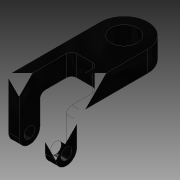
# Autodesk Inventor part: Piston_Holder
Saved by Autodesk Inventor 2015 (Build 190159000, 159)
## iProperties
Created: 2017-02-21
Part Number: Piston_Holder
Material: Acetal Resin, Black
Document SubType Name: Modeling
Designer: Guy
Density: 1.425 g/cm^3
Appearance: Smooth - Black
Author: Guy
Autodesk Inventor part; units mm, degrees
ref_plane "YZ Plane" through (0, 0, 0) normal (1, 0, 0) x (0, 1, 0)
ref_plane "XZ Plane" through (0, 0, 0) normal (0, 1, 0) x (-1, 0, 0)
ref_plane "XY Plane" through (0, 0, 0) normal (0, 0, 1) x (1, 0, 0)
sketch "Sketch1" plane through (0, 0, 0) normal (0, 0, 1) x (1, 0, 0)
  circle A0 centre (0, 0) radius 5
  circle A1 centre (0, 0) radius 9
  line L0 (-9, 0) -> (-9, -35)
  line L1 (9, 0) -> (9, -35)
  line L2 (0, 0) -> (0, -54.7816)
  line L3 (-9, -35) -> (-5, -35)
  line L4 (-5, -35) -> (-5, -15)
  line L5 (5, -15) -> (5, -35)
  line L6 (5, -35) -> (9, -35)
  line L7 (-5, -15) -> (5, -15)
  dimension "d0" = 10
  dimension "d1" = 18
  dimension "d4" = 15
  dimension "d6" = 20
  dimension "d22" = 4
  dimension "d23" = 4
  constraints: 16 end point, 3 coincident, 2 centre point, 2 horizontal, 2 parallel, 2 point on circle, 2 tangent, 1 collinear, 1 perpendicular, 1 point on line, 1 vertical
  measures "d0" diameter of A0
  measures "d1" diameter of A1
  measures "d4" distance from line of L7 point (0, 0)
  measures "d6" distance between parallel lines of L3 L7
  measures "d22" distance between parallel lines of L1 L5
  measures "d23" distance between parallel lines of L0 L4
extrude "Extrusion1" add sketch "Sketch1" along normal blind 23 contours A0 | A1 | L1 L6 L5 L7 L2 A1 | A1 L2 L7 L4 L3 L0
sketch "Sketch2" plane through (9, -35, 0) normal (1, 0, 0) x (0, 0, -1)
  circle A0 centre (-4, 4) radius 2.1
  line L0 (0, 0) -> (0, 35) projected
  line L1 (0, 35) -> (-23, 35) projected
  line L2 (-23, 0) -> (-23, 35) projected
  line L3 (0, 0) -> (-23, 0) projected
  dimension "d9" = 4.2
  dimension "d10" = 4
  dimension "d20" = 4
  constraints: 1 centre point
  measures "d9" diameter of A0
  measures "d10" distance from line of L3 A0.centre
  measures "d20" distance from line of L0 A0.centre
extrude "Extrusion2" cut sketch "Sketch2" against normal through all contours A0
fillet "Fillet1" radius 2 2 edges at (-5, -15, 11.5) (5, -15, 11.5)
sketch "Sketch5" plane through (9, -35, 0) normal (1, 0, 0) x (0, 0, -1)
  circle A0 centre (-4, 4) radius 2.1 projected
  line L0 (0, 0) -> (0, 35) projected
  line L1 (0, 35) -> (-23, 35) projected
  line L2 (-23, 0) -> (-23, 35) projected
  line L3 (0, 0) -> (-23, 0) projected
  line L4 (-23, 20) -> (0, 20) projected
  line L5 (0, 20) -> (-23, 20) projected
  line L6 (-15, 8) -> (0, 8)
  line L7 (0, 8) -> (0, 53.1691)
  line L8 (0, 53.1691) -> (-15, 53.1691)
  line L9 (-15, 53.1691) -> (-15, 8)
  line L10 (0, 0) -> (0, 35) projected
  line L11 (0, 35) -> (0, 35) projected
  line L12 (0, 35) -> (-23, 35) projected
  line L13 (-23, 35) -> (-23, 35) projected
  line L14 (0, 35) -> (-23, 35) projected
  dimension "d28" = 4
  dimension "d29" = 15
  constraints: 8 end point, 2 parallel, 1 horizontal, 1 perpendicular, 1 point on line
  measures "d28" distance from line of A0.centre L6
  measures "d29" distance of L7.end L8.end
extrude "Extrusion5" cut sketch "Sketch5" against normal through all contours L6 L9 L4 L0 | L4 L9 L1 L0 | L1 L9 L8 L7
fillet "Fillet2" radius 4 4 edges at (7, -35, 0) (7, -27, 0) (-7, -27, 0) (-7, -35, 0)
fillet "Fillet3" radius 2 2 edges at (7, -27, 15) (-7, -27, 15)
sketch "Sketch6" plane through (0, 0, 23) normal (0, 0, 1) x (1, 0, 0)
  circle A0 centre (0, 0) radius 5
  dimension "d34" = 10
  constraints: 1 centre point, 1 coincident
  measures "d34" diameter of A0
extrude "Extrusion6" cut sketch "Sketch6" against normal up to next
body "Solid1"
